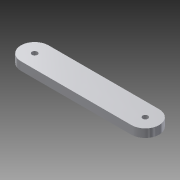
# Autodesk Inventor part: Arm1
Saved by Autodesk Inventor 2015 (Build 190159000, 159)
## iProperties
Created: 2016-11-08
Part Number: Arm1
Material: アルミニウム 6061
Document SubType Name: Modeling
Designer: MobileRoboMaster
Density: 2.7 g/cm^3
Appearance: アルミニウム - フラット
Mass: 478.16 g
Surface Area: 329.115 cm^2
Volume: 177.096 cm^3
Author: MobileRoboMaster
Autodesk Inventor part; units mm, degrees
ref_plane "YZ Plane" through (0, 0, 0) normal (1, 0, 0) x (0, 1, 0)
ref_plane "XZ Plane" through (0, 0, 0) normal (0, 1, 0) x (-1, 0, 0)
ref_plane "XY Plane" through (0, 0, 0) normal (0, 0, 1) x (1, 0, 0)
sketch "スケッチ1" plane through (0, 0, 0) normal (0, 0, 1) x (1, 0, 0)
  line L0 (-100, 25) -> (100, 25)
  line L1 (100, 25) -> (100, -25)
  line L2 (100, -25) -> (-100, -25)
  line L3 (-100, -25) -> (-100, 25)
  arc A0 (-100, 25) -> (-100, -25) centre (-100, 0) ccw
  arc A1 (100, -25) -> (100, 25) centre (100, 0) ccw
  point P0 (0, 0)
  dimension "d0" = 200
  dimension "d1" = 50
  dimension "d2" = 25
  dimension "d3" = 100
  constraints: 8 end point, 4 point on circle, 2 centre point, 2 midpoint, 1 horizontal, 1 parallel
  measures "d0" distance of L0.start L0.end
  measures "d1" distance of L2.end L0.start
  measures "d2" distance from line of L0 point (0, 0)
  measures "d3" distance from line of L3 point (0, 0)
extrude "押し出し1" add sketch "スケッチ1" along normal mid plane 15
sketch "スケッチ2" plane through (0, 0, 7.5) normal (0, 0, 1) x (1, 0, 0)
  line L0 (100, 25) -> (-100, 25) projected
  line L1 (-100, -25) -> (100, -25) projected
  arc A0 (-100, 25) -> (-100, -25) centre (-100, 0) ccw projected
  arc A1 (100, -25) -> (100, 25) centre (100, 0) ccw projected
  circle A2 centre (-100, 0) radius 5
  circle A3 centre (100, 0) radius 5
  point P0 (0, 0)
  dimension "d6" = 10
  dimension "d7" = 10
  constraints: 2 centre point, 2 coincident
  measures "d6" diameter of A2
  measures "d7" diameter of A3
extrude "押し出し2" cut sketch "スケッチ2" against normal through all contours A2 | A3
equation "\"d2\" = 0.5 * d1"
equation "\"d3\" = 0.5 * d0"
